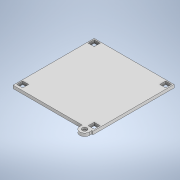
# Autodesk Inventor part: PMS3003_dol
Saved by Autodesk Inventor 2020.3 (Build 243373000, 373)
## iProperties
Created: 2021-02-11
Part Number: PMS3003_dol
Material: Ogólny
Document SubType Name: Modeling
Designer: sitar
Density: 1 g/cm^3
Appearance: Domyślna
Author: sitar
Autodesk Inventor part; units mm, degrees
ref_plane "YZ Plane" through (0, 0, 0) normal (1, 0, 0) x (0, 1, 0)
ref_plane "XZ Plane" through (0, 0, 0) normal (0, 1, 0) x (-1, 0, 0)
ref_plane "XY Plane" through (0, 0, 0) normal (0, 0, 1) x (1, 0, 0)
sketch "Szkic1" plane through (0, 0, 0) normal (0, 1, 0) x (-1, 0, 0)
  line L0 (26.7, -27.1) -> (-26.7, -27.1)
  line L1 (-26.7, -27.1) -> (-26.7, 27.1)
  line L2 (-26.7, 27.1) -> (26.7, 27.1)
  line L3 (26.7, 27.1) -> (26.7, -27.1)
  line L4 (26.7, -27.1) -> (-26.7, 27.1) construction
  line L5 (-26.7, -27.1) -> (26.7, 27.1) construction
  point P0 (0, 0)
  dimension "d0" = 53.4
  dimension "d1" = 54.2
  constraints: 12 end point, 2 midpoint, 2 parallel, 1 horizontal, 1 perpendicular
  measures "d0" distance of L1.end L2.end
  measures "d1" distance of L0.end L1.end
extrude "Wyciągnięcie proste1" add sketch "Szkic1" along normal blind 2
sketch "Szkic11" plane through (0, 2, 0) normal (0, 1, 0) x (1, 0, 0)
  line L0 (-26.7, -27.1) -> (26.7, -27.1) projected
  line L1 (26.7, -27.1) -> (25.9, -27.1)
  line L2 (25.9, -27.1) -> (19.5, -27.1)
  line L3 (19.5, -27.1) -> (19.5, -28.7)
  line L4 (19.5, -28.7) -> (25.9, -28.7)
  line L5 (25.9, -28.7) -> (25.9, -27.1)
  arc A0 (19.5, -28.7) -> (25.9, -28.7) centre (22.7, -28.7) ccw
  point P0 (0, 0)
  dimension "d37" = 0.8
  dimension "d38" = 6.4
  dimension "d39" = 1.6
  dimension "d40" = 3.2
  constraints: 10 end point, 2 parallel, 2 point on circle, 1 centre point, 1 horizontal, 1 perpendicular, 1 point on line
  measures "d37" distance of L0.end L1.end
  measures "d38" distance of L4.end L3.end
  measures "d39" distance of L3.end L2.end
  measures "d40" radius of A0
extrude "Wyciągnięcie proste10" add sketch "Szkic11" against normal blind 2
sketch "Szkic12" plane through (0, 2, 0) normal (0, 1, 0) x (1, 0, 0)
  arc A0 (19.5, -28.7) -> (25.9, -28.7) centre (22.7, -28.7) ccw projected
  circle A1 centre (22.7, -28.7) radius 1.6
  point P0 (0, 0)
  dimension "d43" = 3.2
  constraints: 1 centre point, 1 coincident
  measures "d43" diameter of A1
extrude "Wyciągnięcie proste11" cut sketch "Szkic12" against normal through all
sketch "Szkic49" plane through (0, 0, 0) normal (0, -1, 0) x (1, 0, 0)
  circle A0 centre (22.7, 28.7) radius 1.6 projected
  circle A1 centre (22.7, 28.7) radius 1.6
  point P0 (0, 0)
  constraints: 1 centre point, 1 coincident
extrude "Wyciągnięcie proste41" add sketch "Szkic49" against normal blind 1
sketch "Szkic50" plane through (0, 0, 0) normal (0, -1, 0) x (1, 0, 0)
  circle A0 centre (22.7, 28.7) radius 1.6 projected
  circle A1 centre (22.7, 28.7) radius 1
  point P0 (0, 0)
  dimension "d208" = 2
  constraints: 1 centre point, 1 coincident
  measures "d208" diameter of A1
extrude "Wyciągnięcie proste42" cut sketch "Szkic50" against normal blind 10 contours A1
sketch "Szkic51" plane through (0, 0, 0) normal (0, -1, 0) x (1, 0, 0)
  line L0 (5, -5) -> (-5, -5)
  line L1 (-5, -5) -> (-5, 5)
  line L2 (-5, 5) -> (5, 5)
  line L3 (5, 5) -> (5, -5)
  line L4 (5, -5) -> (-5, 5) construction
  line L5 (-5, -5) -> (5, 5) construction
  point P0 (0, 0)
  dimension "d211" = 10
  dimension "d212" = 10
  constraints: 12 end point, 2 midpoint, 2 parallel, 1 horizontal, 1 perpendicular
  measures "d211" distance of L1.end L2.end
  measures "d212" distance of L0.end L1.end
extrude "Wyciągnięcie proste43" add sketch "Szkic51" along normal blind 1.6
sketch "Szkic52" plane through (0, 2, 0) normal (0, 1, 0) x (1, 0, 0)
  line L0 (-25.9, 26.3) -> (-21.9, 26.3)
  line L1 (-21.9, 26.3) -> (-21.9, 22.3)
  line L2 (-21.9, 22.3) -> (-25.9, 22.3)
  line L3 (-25.9, 22.3) -> (-25.9, 26.3)
  line L4 (21.9, 26.3) -> (25.9, 26.3)
  line L5 (25.9, 26.3) -> (25.9, 22.3)
  line L6 (25.9, 22.3) -> (21.9, 22.3)
  line L7 (21.9, 22.3) -> (21.9, 26.3)
  line L8 (-25.9, -21.5) -> (-21.9, -21.5)
  line L9 (-21.9, -21.5) -> (-21.9, -25.5)
  line L10 (-21.9, -25.5) -> (-25.9, -25.5)
  line L11 (-25.9, -25.5) -> (-25.9, -21.5)
  line L12 (21.9, -21.5) -> (25.9, -21.5)
  line L13 (25.9, -21.5) -> (25.9, -25.5)
  line L14 (25.9, -25.5) -> (21.9, -25.5)
  line L15 (21.9, -25.5) -> (21.9, -21.5)
  line L16 (-25.9, 26.3) -> (-26.7, 26.3)
  line L17 (-25.9, -21.5) -> (-26.7, -21.5)
  line L18 (25.9, 26.3) -> (26.7, 26.3)
  line L19 (25.9, -21.5) -> (26.7, -21.5)
  line L20 (26.7, -27.1) -> (26.7, 27.1) projected
  line L21 (-26.7, 27.1) -> (-26.7, -27.1) projected
  line L22 (-25.9, 26.3) -> (-25.9, 27.1)
  line L23 (25.9, 26.3) -> (25.9, 27.1)
  line L24 (26.7, -27.1) -> (26.7, 27.1) projected
  line L25 (25.9, 26.3) -> (26.7, 26.3) construction
  line L26 (26.7, 27.1) -> (-26.7, 27.1) projected
  line L27 (-25.9, -25.5) -> (-25.9, -27.1)
  line L28 (-26.7, 27.1) -> (-26.7, -27.1) projected
  line L29 (-25.9, -25.5) -> (-24.3, -25.5) construction
  line L30 (25.9, -25.5) -> (25.9, -27.1)
  line L31 (-26.7, -27.1) -> (19.5, -27.1) projected
  point P0 (0, 0)
  dimension "d215" = 4
  dimension "d216" = 4
  dimension "d217" = 4
  dimension "d218" = 4
  dimension "d219" = 4
  dimension "d220" = 4
  dimension "d221" = 4
  dimension "d222" = 4
  dimension "d223" = 0.8
  dimension "d224" = 0.8
  dimension "d225" = 0.8
  dimension "d226" = 0.8
  dimension "d227" = 0.8
  dimension "d228" = 0.8
  dimension "d229" = 90
  dimension "d230" = 1.6
  dimension "d231" = 90
  dimension "d232" = 1.6
  constraints: 52 end point, 10 horizontal, 10 parallel, 8 point on line, 6 perpendicular, 2 vertical
  measures "d215" distance of L1.end L2.end
  measures "d216" distance of L0.end L1.end
  measures "d217" distance of L5.end L6.end
  measures "d218" distance of L4.end L5.end
  measures "d219" distance of L9.end L10.end
  measures "d220" distance of L8.end L9.end
  measures "d221" distance of L13.end L14.end
  measures "d222" distance of L12.end L13.end
  measures "d223" distance of L0.start L16.end
  measures "d224" distance of L8.start L17.end
  measures "d225" distance of L4.end L18.end
  measures "d226" distance of L12.end L19.end
  measures "d227" distance of L0.start L22.end
  measures "d228" distance of L4.end L23.end
  measures "d229" angle of L25 L23
  measures "d230" distance of L10.end L27.end
  measures "d231" angle of L27 L29
  measures "d232" distance of L13.end L30.end
extrude "Wyciągnięcie proste44" cut sketch "Szkic52" against normal up to surface (2 mm away) contours L0 L1 L2 L3 | L13 L14 L15 L12 | L5 L6 L7 L4 | L8 L9 L10 L11
